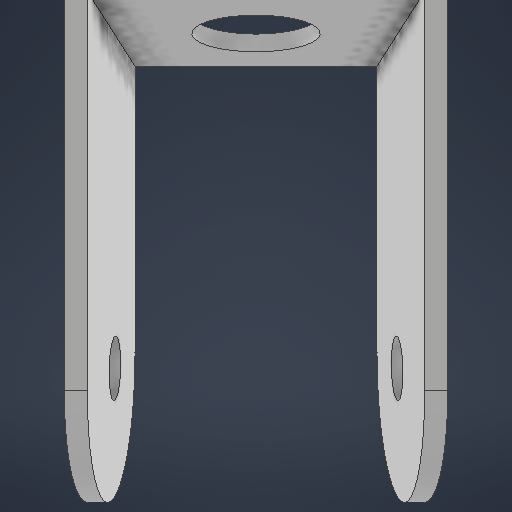
# Autodesk Inventor part: Part1
Saved by Autodesk Inventor 2026 (Build 300175050, 175E)
## iProperties
Created: 2026-05-07
Part Number: Part1
Material: Generic
Document SubType Name: Modeling
Designer: Administrator
Density: 1 g/cm^3
Appearance: Default
Author: Administrator
Autodesk Inventor part; units mm, degrees
ref_plane "YZ Plane" through (0, 0, 0) normal (1, 0, 0) x (0, 1, 0)
ref_plane "XZ Plane" through (0, 0, 0) normal (0, 1, 0) x (-1, 0, 0)
ref_plane "XY Plane" through (0, 0, 0) normal (0, 0, 1) x (1, 0, 0)
sketch "Sketch1" plane through (0, 0, 0) normal (0, 1, 0) x (-1, 0, 0)
  line L0 (50, 0) -> (50, 75)
  line L1 (50, 75) -> (0, 75)
  line L2 (0, 75) -> (0, 0)
  line L3 (3, 0) -> (3, 72)
  line L4 (3, 72) -> (47, 72)
  line L5 (47, 72) -> (47, 0)
  line L6 (0, 0) -> (3, 0)
  line L7 (47, 0) -> (50, 0)
  dimension "d0" = 50
  dimension "d1" = 75
  dimension "d2" = 3
  constraints: 16 end point, 4 perpendicular, 1 collinear, 1 horizontal, 2 other
  measures "d0" distance of L2.end L0.start
  measures "d1" distance of L0.start L0.end
  measures "d2" distance between parallel lines of L1 L4
extrude "Extrusion1" add sketch "Sketch1" along normal mid plane 40
fillet "Fillet1" radius 20 4 edges at (-48.5, 20, 0) (-48.5, -20, 0) (-1.5, 20, 0) (-1.5, -20, 0)
fillet "Fillet2" radius 3 2 edges at (-50, 0, 75) (0, 0, 75)
sketch "Sketch2" plane through (-50, 0, 20) normal (-1, 0, 0) x (0, 0, 1)
  circle A0 centre (0, 0) radius 5
  point P0 (-20, 0)
  dimension "d7" = 10
  constraints: 1 centre point
  measures "d7" diameter of A0
extrude "Extrusion2" cut sketch "Sketch2" against normal through all
sketch "Sketch3" plane through (-47, 20, 75) normal (0, 0, 1) x (1, 0, 0)
  circle A0 centre (22, -20) radius 10
  point P0 (47, -20)
  dimension "d10" = 20
  constraints: 1 centre point
  measures "d10" diameter of A0
extrude "Extrusion3" cut sketch "Sketch3" against normal blind 10
body "Solid1"
